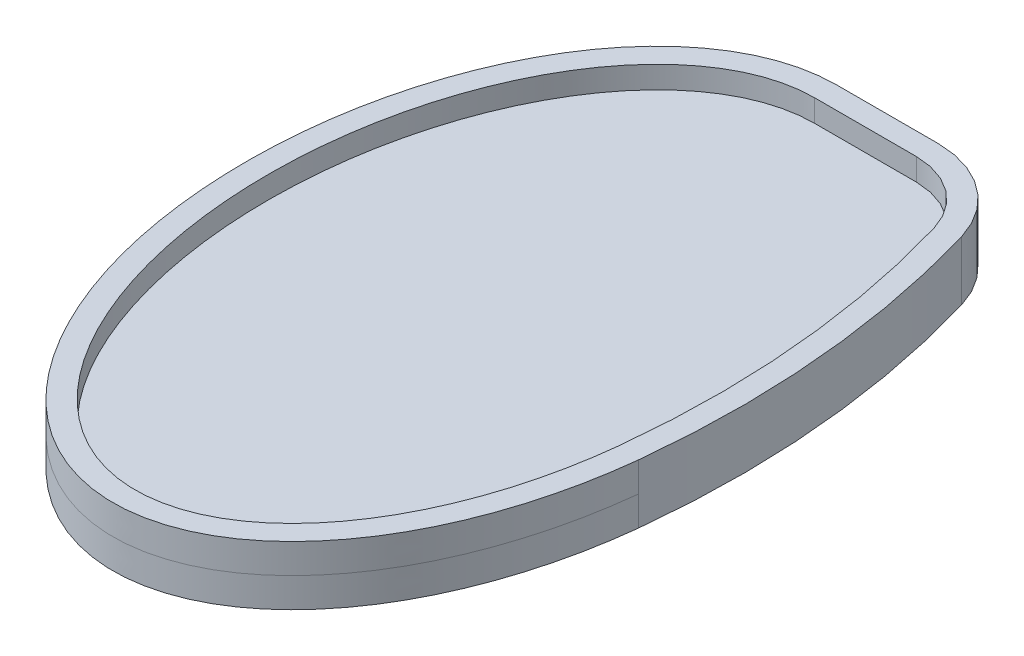
# Autodesk Inventor part: chip_lid
Saved by Autodesk Inventor 2022 (Build 260153070, 153G)
## iProperties
Created: 2022-04-02
Part Number: chip_lid
Material: Generic
Document SubType Name: Modeling
Designer: a laptop
Density: 1 g/cm^3
Appearance: Default
Author: a laptop
Autodesk Inventor part; units mm, degrees
ref_plane "YZ Plane" through (0, 0, 0) normal (1, 0, 0) x (0, 1, 0)
ref_plane "XZ Plane" through (0, 0, 0) normal (0, 1, 0) x (-1, 0, 0)
ref_plane "XY Plane" through (0, 0, 0) normal (0, 0, 1) x (1, 0, 0)
sketch "Sketch1" plane through (0, 0, 0) normal (0, 1, 0) x (-1, 0, 0)
  ellipse E0 centre (0, 0) end of major axis (-28, 0) minor radius 46
  line L0 (0, -46) -> (-13.7715, -46)
  arc A0 (-27.5646, 8.0806) -> (-23.3629, -38.8294) centre (91.7338, -4.877) ccw
  arc A1 (-23.3629, -38.8294) -> (-13.7715, -46) centre (-13.7715, -36) ccw
  point P0 (-21, -46)
  dimension "d0" = 28
  dimension "d1" = 46
  dimension "d3" = 120
  dimension "d5" = 21
  dimension "d6" = 10
  constraints: 5 point on circle, 2 centre point, 2 end point, 2 tangent, 1 coincident, 1 horizontal, 1 point on line, 1 vertical alignment, 5 other
  measures "d3" radius of A0
  measures "d5" distance of L0.start point (-21, -46)
  measures "d6" radius of A1
extrude "Extrusion1" add sketch "Sketch1" against normal blind 4
thicken "Thicken1" operation add thickness 3 both sides no extend neighbours yes toward (-0.9993547, 0, 0.0359184) faces at (-27.9513, -2.6667, 2.7114) (26.8244, -2.6667, -23.4231) (23.1369, -1.3333, -39.5057) (9.181, -2.6667, -46)
extrude "Extrusion2" cut sketch "Sketch1" against normal blind 3
mirror "Mirror1" about plane through (0.1331, -4, 0) normal (0, -1, 0) of "Extrusion1", "Thicken1", "Extrusion2"
body "Solid1"
